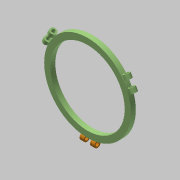
# Autodesk Inventor part: EndEffector
Saved by Autodesk Inventor 2015 (Build 190159000, 159)
## iProperties
Created: 2016-06-12
Part Number: EndEffector
Material: 一般
Document SubType Name: Modeling
Designer: kumagai
Density: 1 g/cm^3
Appearance: 既定(1)
Author: kumagai
Autodesk Inventor part; units mm, degrees
ref_plane "YZ Plane" through (0, 0, 0) normal (1, 0, 0) x (0, 1, 0)
ref_plane "XZ Plane" through (0, 0, 0) normal (0, 1, 0) x (-1, 0, 0)
ref_plane "XY Plane" through (0, 0, 0) normal (0, 0, 1) x (1, 0, 0)
sketch "スケッチ1" plane through (0, 0, 0) normal (0, 1, 0) x (-1, 0, 0)
  circle A0 centre (0, 0) radius 70
  circle A1 centre (0, 0) radius 60
  dimension "d0" = 140
  dimension "d1" = 120
  constraints: 2 centre point, 2 coincident
  measures "d0" diameter of A0
  measures "d1" diameter of A1
extrude "押し出し1" add sketch "スケッチ1" along normal mid plane 8
sketch "スケッチ2" plane through (0, 0, 0) normal (0, 1, 0) x (-1, 0, 0)
  line L0 (12, -78) -> (5, -78)
  line L1 (5, -78) -> (5, -80)
  line L2 (5, -80) -> (12, -80)
  line L3 (12, -80) -> (12, -78)
  line L4 (-5, -78) -> (-12, -78)
  line L5 (-12, -78) -> (-12, -80)
  line L6 (-12, -80) -> (-5, -80)
  line L7 (-5, -80) -> (-5, -78)
  line L8 (0, -109.632) -> (0, 99.9387) projected
  line L9 (-98, 0) -> (98, 0) projected
  line L10 (18.6629, -75) -> (-18.486, -75)
  point P0 (0, 0)
  dimension "d5" = 75
  dimension "d6" = 3
  dimension "d7" = 5
  dimension "d8" = 10
  dimension "d9" = 24
  constraints: 18 end point, 4 parallel, 3 horizontal, 2 perpendicular, 2 point on line, 2 other
  measures "d5" distance from line of L9 L10.start
  measures "d6" distance between parallel lines of L10 L0
  measures "d7" distance between parallel lines of L10 L2
  measures "d8" distance between parallel lines of L7 L1
  measures "d9" distance between parallel lines of L3 L5
revolve "回転1" add sketch "スケッチ2" angle 360 about axis through (-18.6629, 0, -75) along (1, 0, 0)
pattern_circular "円形状パターン1" count 3 over 360 about axis through (0, -10, 0) along (0, 1, 0) of "回転1"
